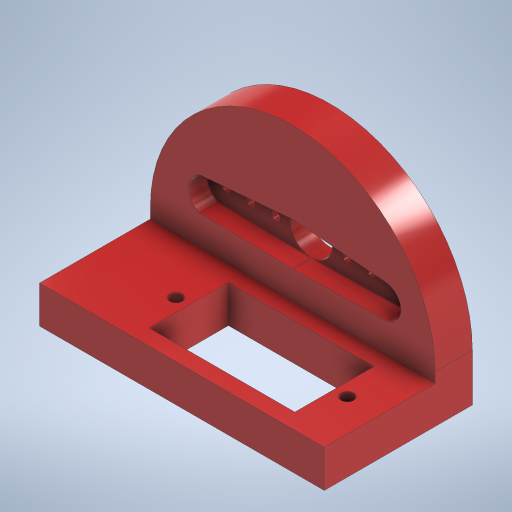
# Autodesk Inventor part: unions1s2
Saved by Autodesk Inventor 2024.3 (Build 283343000, 343)
## iProperties
Created: 2025-08-12
Part Number: unions1s2
Material: Generic
Document SubType Name: Modeling
Designer: jscme
Density: 1 g/cm^3
Appearance: Default
Author: jscme
Autodesk Inventor part; units mm, degrees
note: some values were not read from the file. Chosen so that the rebuilt part matches the saved one: arc direction of "Extrusion4"; arc direction of "Extrusion5".
ref_plane "YZ Plane" through (0, 0, 0) normal (1, 0, 0) x (0, 1, 0)
ref_plane "XZ Plane" through (0, 0, 0) normal (0, 1, 0) x (-1, 0, 0)
ref_plane "XY Plane" through (0, 0, 0) normal (0, 0, 1) x (1, 0, 0)
sketch "Sketch1" plane through (0, 0, 0) normal (0, 1, 0) x (-1, 0, 0)
  line L0 (22.86, 8.89) -> (-22.86, 8.89)
  line L1 (-22.86, 8.89) -> (-22.86, -8.89)
  line L2 (-22.86, -8.89) -> (22.86, -8.89)
  line L3 (22.86, -8.89) -> (22.86, 8.89)
  point P0 (0, 0)
  point P1 (0, -8.89)
  point P2 (22.86, 0)
  dimension "d0" = 45.72
  dimension "d1" = 17.78
  constraints: 8 end point, 2 midpoint, 2 parallel, 1 horizontal, 1 horizontal alignment, 1 perpendicular, 1 vertical alignment
  measures "d0" distance of L1.end L2.end
  measures "d1" distance of L0.end L1.end
extrude "Extrusion1" add sketch "Sketch1" along normal blind 6
sketch "Sketch2" plane through (0, 6, 0) normal (0, 1, 0) x (1, 0, 0)
  line L0 (-7.7772, -6.35) -> (15.5908, -6.35)
  line L1 (15.5908, -6.35) -> (15.5908, 6.35)
  line L2 (15.5908, 6.35) -> (-7.7772, 6.35)
  line L3 (-7.7772, 6.35) -> (-7.7772, -6.35)
  circle A0 centre (-9.86, 0) radius 1.016
  circle A1 centre (17.6736, 0) radius 1.016
  line L4 (-22.86, 8.89) -> (-22.86, -8.89) projected
  line L5 (22.86, 8.89) -> (-22.86, 8.89) projected
  point P0 (3.9068, 0)
  point P1 (-7.7772, 0)
  point P2 (3.9068, 6.35)
  dimension "d4" = 23.368
  dimension "d5" = 12.7
  dimension "d6" = 2.032
  dimension "d7" = 2.032
  dimension "d8" = 2.0828
  dimension "d9" = 2.0828
  dimension "d34" = 13
  dimension "d35" = 2.54
  constraints: 8 end point, 3 horizontal alignment, 2 centre point, 2 midpoint, 2 parallel, 1 horizontal, 1 perpendicular, 1 vertical alignment
  measures "d4" distance of L1.end L2.end
  measures "d5" distance of L2.end L0.start
  measures "d6" diameter of A0
  measures "d7" diameter of A1
  measures "d8" distance from line of L3 A0.centre
  measures "d9" distance from line of L1 A1.centre
  measures "d34" distance from line of L4 A0.centre
  measures "d35" distance between parallel lines of L5 L2
extrude "Extrusion2" cut sketch "Sketch2" against normal blind 15
sketch "Sketch3" plane through (22.86, 0, -8.89) normal (0, 0, -1) x (-1, 0, 0)
  line L0 (0, 0) -> (45.72, 0) projected
  circle A0 centre (22.86, 13.97) radius 3.429
  line L1 (22.86, 17.399) -> (7.9031, 16.12)
  line L2 (22.86, 10.541) -> (7.8514, 10.8324)
  arc A1 (7.9031, 16.12) -> (7.8514, 10.8324) centre (8.1294, 13.4738) ccw
  arc A2 (37.8686, 10.8324) -> (37.8169, 16.12) centre (36.641, 13.4645) ccw
  line L3 (22.86, 17.399) -> (37.8169, 16.12)
  line L4 (22.86, 10.541) -> (37.8686, 10.8324)
  line L5 (45.72, 0) -> (45.72, 6) projected
  line L6 (45.72, 0) -> (45.72, 7.62)
  line L7 (0, 0) -> (0, 7.62)
  arc A3 (45.72, 7.62) -> (0, 7.62) centre (22.86, 7.62) ccw
  point P0 (22.86, 0)
  point P1 (22.7269, 10.5436)
  point P2 (22.9931, 10.5436)
  point P3 (22.2778, 17.3492)
  point P4 (23.4422, 17.3492)
  point P5 (22.86, 30.48)
  point P6 (39.5451, 13.4929)
  dimension "d14" = 6
  dimension "d15" = 6.858
  dimension "d25" = 7.62
  dimension "d30" = 6
  dimension "d31" = 16.51
  dimension "d33" = 13.781
  constraints: 12 end point, 10 point on circle, 4 centre point, 3 tangent, 3 vertical alignment, 1 collinear, 1 equal length, 1 vertical
  measures "d14" angle of L2 L1
  measures "d15" diameter of A0
  measures "d25" distance of L0.end L6.end
  measures "d30" angle of L3 L4
  measures "d31" distance of point (22.86, 30.48) A0.centre
  measures "d33" horizontal distance of A2.centre A0.centre
extrude "Extrusion3" add sketch "Sketch3" along normal blind 3 contours A0 L1 L3 | L2 A1 L1 A0 | A0 L3 A2 L4 | L3 A0
extrude "Extrusion6" add sketch "Sketch3" along normal blind 6 contours L7 A3 L6 L5 L0 | A0 L1 L3 | L2 A1 L1 A0 | A0 L3 A2 L4 | A0 L1 | L3 A0
extrude "Extrusion4" cut sketch "Sketch3" along normal through all contours A0 L1 L3 | A0 L1 | L3 A0
extrude "Extrusion5" cut sketch "Sketch3" along normal blind 3 contours A0 L1 L3 | L2 A1 L1 A0 | A0 L3 A2 L4 | A0 L1 | L3 A0
sketch "Sketch4" plane through (22.86, 0, -8.89) normal (0, 0, 1) x (1, 0, 0)
  line L0 (-22.86, 19.9111) -> (-22.86, 7.8054)
  circle A0 centre (-32.5451, 13.4929) radius 0.75
  circle A1 centre (-36.5451, 13.4929) radius 0.75
  circle A2 centre (-28.5451, 13.4929) radius 0.75
  arc A3 (-37.8169, 16.12) -> (-37.8686, 10.8324) centre (-36.641, 13.4645) ccw projected
  circle A4 centre (-17.1749, 13.4929) radius 0.75
  circle A5 centre (-13.1749, 13.4929) radius 0.75
  circle A6 centre (-9.1749, 13.4929) radius 0.75
  point P0 (-22.86, 0)
  point P1 (-36.7619, 13.4929)
  point P2 (-39.5451, 13.4929)
  point P3 (-39.5451, 13.4929)
  point P4 (-9.079, 13.4645)
  dimension "d54" = 1.5
  dimension "d55" = 1.5
  dimension "d56" = 1.5
  dimension "d57" = 4
  dimension "d58" = 4
  dimension "d59" = 3
  constraints: 6 centre point, 4 horizontal alignment, 4 symmetric about line, 2 end point, 2 point on circle, 1 vertical, 3 other
  measures "d54" diameter of A1
  measures "d55" diameter of A0
  measures "d56" diameter of A2
  measures "d57" distance of A1.centre A0.centre
  measures "d58" distance of A0.centre A2.centre
  measures "d59" distance of point (-39.545, 13.493) A1.centre
extrude "Extrusion7" cut sketch "Sketch4" against normal blind 4
body "Solid1"
